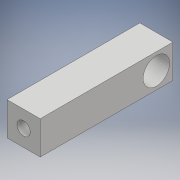
# Autodesk Inventor part: SupportBarreCodeuse
Saved by Autodesk Inventor 2017 SP1 (Build 210196100, 196)
## iProperties
Part Number: SupportBarreCodeuse
Material: Générique
Document SubType Name: Modeling
Designer: Sylvain
Density: 1 g/cm^3
Appearance: Par défaut
Author: Sylvain
Autodesk Inventor part; units mm, degrees
ref_plane "YZ Plane" through (0, 0, 0) normal (1, 0, 0) x (0, 1, 0)
ref_plane "XZ Plane" through (0, 0, 0) normal (0, 1, 0) x (-1, 0, 0)
ref_plane "XY Plane" through (0, 0, 0) normal (0, 0, 1) x (1, 0, 0)
sketch "Esquisse1" plane through (0, 0, 0) normal (0, 1, 0) x (-1, 0, 0)
  line L0 (0, 0) -> (10, 0)
  line L1 (10, 0) -> (10, -10)
  line L2 (10, -10) -> (0, -10)
  line L3 (0, -10) -> (0, 0)
  dimension "d0" = 10
  dimension "d1" = 10
  constraints: 8 end point, 2 parallel, 1 horizontal, 1 perpendicular
  measures "d0" distance of L2.end L0.start
  measures "d1" distance of L1.end L2.end
extrude "Extrusion1" add sketch "Esquisse1" along normal blind 40
sketch "Esquisse2" plane through (0, 0, 0) normal (1, 0, 0) x (0, 0, -1)
  line L0 (10, 0) -> (0, 0) projected
  line L1 (0, 0) -> (0, 40) projected
  point P0 (5, 35)
  dimension "d4" = 35
  dimension "d5" = 5
  measures "d4" distance from line of L0 point (5, 35)
  measures "d5" distance from line of L1 point (5, 35)
hole "Perçage1" at (0, 35, -5) direction (-1, 0, 0) diameter 8 depth 10 tip angle 118
sketch "Esquisse3" plane through (0, 0, 0) normal (0, -1, 0) x (1, 0, 0)
  line L0 (-10, 0) -> (0, 0) projected
  line L1 (-10, 0) -> (-10, -10) projected
  point P0 (-5, -5)
  dimension "d13" = 5
  dimension "d14" = 5
  measures "d13" distance from line of L0 point (-5, -5)
  measures "d14" distance from line of L1 point (-5, -5)
hole "Perçage2" at (-5, 0, -5) direction (0, 1, 0) diameter 4 depth 25 tip angle 118
